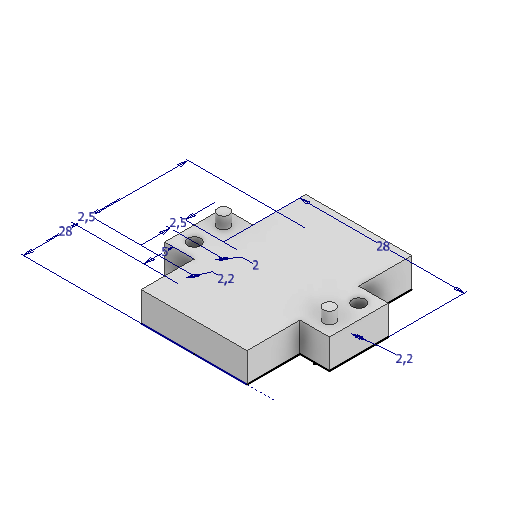
# Autodesk Inventor part: SupportoSopra
Saved by Autodesk Inventor 2025.4 (Build 294407000, 407)
## iProperties
Created: 2026-04-22
Part Number: SupportoSopra
Material: Generic
Document SubType Name: Modeling
Designer: gdira
Density: 1 g/cm^3
Appearance: Default
Author: gdira
Autodesk Inventor part; units mm, degrees
ref_plane "YZ Plane" through (0, 0, 0) normal (1, 0, 0) x (0, 1, 0)
ref_plane "XZ Plane" through (0, 0, 0) normal (0, 1, 0) x (-1, 0, 0)
ref_plane "XY Plane" through (0, 0, 0) normal (0, 0, 1) x (1, 0, 0)
sketch "Sketch1" plane through (0, 0, 0) normal (0, 1, 0) x (-1, 0, 0)
  line L0 (5, -28) -> (23, -28)
  line L1 (23, 0) -> (5, 0)
  line L2 (0, 0) -> (23, 0) construction
  line L3 (5, -5) -> (5, -23)
  line L4 (28, -9) -> (28, -14)
  line L5 (23, -12) -> (23, -9)
  line L6 (23, -9) -> (28, -9)
  line L7 (28, -19) -> (28, -14)
  line L8 (23, -14) -> (23, -19)
  line L9 (23, -19) -> (28, -19)
  line L10 (23, -3) -> (23, -23)
  line L11 (28, -19) -> (28, -14)
  line L12 (28, -14) -> (28, -9)
  line L13 (28, -9) -> (28, -14)
  line L14 (28, -14) -> (28, -19)
  line L15 (23, -23) -> (23, -28)
  line L16 (23, -3) -> (23, 0)
  line L17 (14, -28) -> (14, 0)
  line L18 (5, -3) -> (5, -23)
  line L19 (0, -19) -> (0, -14)
  line L20 (5, -14) -> (5, -19)
  line L21 (5, -19) -> (0, -19)
  line L22 (0, -9) -> (0, -14)
  line L23 (5, -12) -> (5, -9)
  line L24 (5, -9) -> (0, -9)
  line L25 (0, -19) -> (0, -14)
  line L26 (0, -14) -> (0, -9)
  line L27 (0, -9) -> (0, -14)
  line L28 (0, -14) -> (0, -19)
  circle A0 centre (2.5, -16.5) radius 1.1
  circle A1 centre (2.5, -11.5) radius 1
  line L29 (5, -23) -> (5, -28)
  line L30 (5, 0) -> (5, -28)
  line L31 (25.5, -16.5) -> (28, -16.5)
  line L32 (25.5, -11.5) -> (28, -11.5)
  circle A2 centre (25.5, -16.5) radius 1
  circle A3 centre (25.5, -11.5) radius 1.1
  point P0 (25.5, -19)
  point P1 (25.5, -9)
  point P2 (23, -28)
  point P3 (23, 0)
  point P4 (23, -28)
  point P5 (23, 0)
  point P6 (2.5, -19)
  point P7 (2.5, -9)
  dimension "d18" = 5
  dimension "d20" = 2.5
  dimension "d22" = 2.5
  dimension "d25" = 2
  dimension "d26" = 2.2
  dimension "d27" = 2.2
  dimension "d28" = 28
  dimension "d29" = 28
  constraints: 66 end point, 14 symmetric about line, 5 midpoint, 4 centre point, 3 perpendicular, 3 point on line, 2 coincident, 1 horizontal, 1 parallel
  measures "d18" distance of L4.start L4.end
  measures "d20" distance of point (25.5, -19) L31.start
  measures "d22" distance of point (25.5, -9) L32.start
  measures "d25" diameter of A2
  measures "d26" diameter of A3
  measures "d27" diameter of A0
  measures "d28" distance between parallel lines of L19 L7
  measures "d29" distance between parallel lines of L1 L0
extrude "Extrusion4" add sketch "Sketch1" along normal blind 5
extrude "Extrusion5" add sketch "Sketch1" along normal blind 7 contours A1 | A2
extrude "Extrusion6" add sketch "Sketch1" along normal blind 2.8 contours A0 | A3
body "Solid2"
